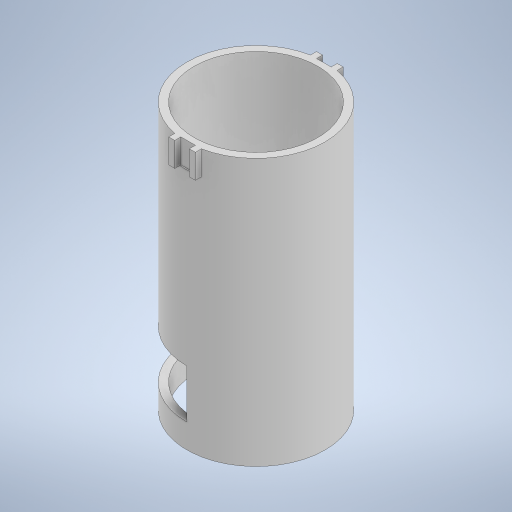
# Autodesk Inventor part: VerticalShaft
Saved by Autodesk Inventor 2024.3 (Build 283343000, 343)
## iProperties
Created: 2025-02-25
Part Number: VerticalShaft
Material: Generic
Document SubType Name: Modeling
Designer: ajclo
Density: 1 g/cm^3
Appearance: Default
Author: ajclo
Autodesk Inventor part; units mm, degrees
ref_plane "YZ Plane" through (0, 0, 0) normal (1, 0, 0) x (0, 1, 0)
ref_plane "XZ Plane" through (0, 0, 0) normal (0, 1, 0) x (-1, 0, 0)
ref_plane "XY Plane" through (0, 0, 0) normal (0, 0, 1) x (1, 0, 0)
sketch "Sketch1" plane through (0, 0, 0) normal (0, 1, 0) x (-1, 0, 0)
  circle A0 centre (0, 0) radius 57
  circle A1 centre (0, 0) radius 51
  dimension "d0" = 114
  dimension "d1" = 102
  constraints: 2 centre point, 2 coincident
  measures "d0" diameter of A0
  measures "d1" diameter of A1
extrude "Extrusion1" add sketch "Sketch1" along normal blind 220
sketch "Sketch2" plane through (0, 220, 0) normal (0, 1, 0) x (1, 0, 0)
  circle A0 centre (0, 0) radius 57 projected
  line L0 (-11, -55.9285) -> (11, -55.9285)
  line L1 (11, -55.9285) -> (11, 55.9285)
  line L2 (11, 55.9285) -> (-11, 55.9285)
  line L3 (-11, 55.9285) -> (-11, -55.9285)
  line L4 (-11, -55.9285) -> (11, 55.9285) construction
  line L5 (11, -55.9285) -> (-11, 55.9285) construction
  circle A1 centre (0, 0) radius 57 projected
  dimension "d19" = 21.9999
  constraints: 12 end point, 2 midpoint, 2 parallel, 1 horizontal, 1 perpendicular, 1 point on circle
  measures "d19" distance of L1.end L2.end
extrude "Extrusion2" cut sketch "Sketch2" against normal blind 20 contours L2 A0 | A0 L0
ref_plane "Work Plane1" through (0, 200, 0) normal (0, 1, 0) x (1, 0, 0)
sketch "Sketch3" plane through (0, 200, 0) normal (0, 1, 0) x (1, 0, 0)
  line L0 (11, 55.9285) -> (-11, 55.9285) projected
  line L1 (11, 55.9285) -> (6, 55.9285)
  line L2 (6, 55.9285) -> (6, 60.9285)
  line L3 (6, 60.9285) -> (11, 60.9285)
  line L4 (11, 60.9285) -> (11, 55.9285)
  point P0 (0, 0)
  dimension "d7" = 5
  dimension "d8" = 5
  constraints: 8 end point, 2 parallel, 1 horizontal, 1 perpendicular
  measures "d7" distance of L2.end L3.end
  measures "d8" distance of L3.end L0.start
extrude "Extrusion3" add sketch "Sketch3" along normal blind 20
mirror "Mirror1" about plane through (0, 0, 0) normal (1, 0, 0) of "Extrusion3"
mirror "Mirror2" about plane through (0, 0, 0) normal (0, 0, 1) of "Extrusion3", "Mirror1"
sketch "Sketch4" plane through (0, 0, 0) normal (1, 0, 0) x (0, 1, 0)
  line L0 (0, -57) -> (200, -57) projected
  line L1 (0, 57) -> (200, 57) projected
  line L2 (20, -57) -> (60, -57)
  line L3 (60, -57) -> (60, 57)
  line L4 (60, 57) -> (20, 57)
  line L5 (20, 57) -> (20, -57)
  line L6 (220, 51) -> (0, 51) projected
  line L7 (220, -51) -> (0, -51) projected
  line L8 (22, 51) -> (58, 51)
  line L9 (58, 51) -> (58, -51)
  line L10 (58, -51) -> (22, -51)
  line L11 (22, -51) -> (22, 51)
  line L12 (0, -57) -> (0, 57) projected
  point P0 (0, 0)
  dimension "d11" = 40
  dimension "d12" = 36
  dimension "d13" = 2
  dimension "d14" = 20
  constraints: 16 end point, 4 parallel, 4 point on line, 2 horizontal, 2 perpendicular
  measures "d11" distance between parallel lines of L5 L3
  measures "d12" distance between parallel lines of L11 L9
  measures "d13" distance between parallel lines of L5 L11
  measures "d14" distance between parallel lines of L12 L5
extrude "Extrusion4" cut sketch "Sketch4" against normal through all contours L5 L7 L3 L0 | L5 L6 L11 L7 | L7 L9 L6 L3 | L5 L1 L3 L6 | L11 L6 L9 L7
body "Solid1"
